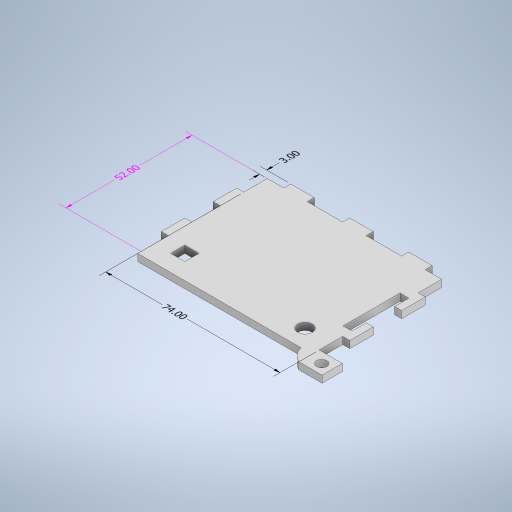
# Autodesk Inventor part: Parede_lateral_2
Saved by Autodesk Inventor 2024 (Build 280153000, 153)
## iProperties
Created: 2023-11-29
Part Number: Parede_lateral_2
Material: Genérico
Document SubType Name: Modeling
Designer: caiot
Density: 1 g/cm^3
Appearance: Padrão
Author: caiot
Autodesk Inventor part; units mm, degrees
ref_plane "YZ Plane" through (0, 0, 0) normal (1, 0, 0) x (0, 1, 0)
ref_plane "XZ Plane" through (0, 0, 0) normal (0, 1, 0) x (-1, 0, 0)
ref_plane "XY Plane" through (0, 0, 0) normal (0, 0, 1) x (1, 0, 0)
sketch "Esboço1" plane through (0, 0, 0) normal (0, 1, 0) x (-1, 0, 0)
  line L0 (0, 0) -> (-74, 0)
  line L1 (-74, 0) -> (-74, -52)
  line L2 (-74, -52) -> (0, -52)
  line L3 (0, -52) -> (0, 0)
  line L4 (-6.0465, -39.0348) -> (-22.7965, -39.0348)
  line L5 (-22.7965, -39.0348) -> (-22.7965, -36.6698)
  line L6 (-22.7965, -36.6698) -> (-6.0465, -36.6698)
  line L7 (-6.0465, -36.6698) -> (-6.0465, -39.0348)
  dimension "d0" = 74
  dimension "d1" = 52
  dimension "d22" = 16.75
  dimension "d23" = 2.365
  constraints: 16 end point, 4 parallel, 2 horizontal, 2 perpendicular
  measures "d0" distance of L2.end L1.end
  measures "d1" distance of L1.end L0.end
  measures "d22" distance of L5.end L6.end
  measures "d23" distance of L4.end L5.end
extrude "Extrusão1" add sketch "Esboço1" along normal blind 3 contours L3 L2 L1 L0 | L4 L5 L6 L7
sketch "Esboço2" plane through (0, 3, 0) normal (0, 1, 0) x (1, 0, 0)
  line L0 (0, 52) -> (0, 0) projected
  line L1 (74, 52) -> (0, 52) projected
  line L2 (7, 52) -> (17, 52)
  line L3 (17, 52) -> (17, 55)
  line L4 (17, 55) -> (7, 55)
  line L5 (7, 55) -> (7, 52)
  line L6 (32, 52) -> (42, 52)
  line L7 (42, 52) -> (42, 55)
  line L8 (42, 55) -> (32, 55)
  line L9 (32, 55) -> (32, 52)
  line L10 (57, 52) -> (67, 52)
  line L11 (67, 52) -> (67, 55)
  line L12 (67, 55) -> (57, 55)
  line L13 (57, 55) -> (57, 52)
  line L14 (74, 0) -> (74, 52) projected
  point P0 (17, 52)
  point P1 (67, 52)
  point P2 (42, 52)
  point P3 (7, 53.5)
  point P4 (67, 53.5)
  point P5 (57, 53.5)
  point P6 (42, 53.5)
  point P7 (17, 53.5)
  point P8 (32, 53.5)
  point P9 (0, 26)
  dimension "d13" = 3
  dimension "d38" = 7
  dimension "d39" = 7
  dimension "d40" = 15
  dimension "d42" = 10
  dimension "d44" = 10
  dimension "d45" = 10
  constraints: 24 end point, 7 midpoint, 6 parallel, 5 point on line, 3 horizontal, 3 perpendicular
  measures "d13" distance of L3.end L2.end
  measures "d38" distance from line of L0 point (7, 53.5)
  measures "d39" distance from line of L14 point (67, 53.5)
  measures "d40" distance of point (57, 53.5) point (42, 53.5)
  measures "d42" distance from line of point (17, 53.5) L5
  measures "d44" distance of point (67, 53.5) point (57, 53.5)
  measures "d45" distance of point (32, 53.5) point (42, 53.5)
extrude "Extrusão2" add sketch "Esboço2" against normal blind 3
sketch "Esboço5" plane through (0, 3, 0) normal (0, 1, 0) x (1, 0, 0)
  circle A0 centre (63, 5) radius 3.1
  line L0 (0, 52) -> (0, 0) projected
  line L1 (7, 52) -> (0, 52) projected
  line L2 (74, 0) -> (74, 52) projected
  line L3 (0, 0) -> (74, 0) projected
  point P0 (3.5, 52)
  dimension "d46" = 6.2
  dimension "d113" = 11
  dimension "d114" = 52
  dimension "d116" = 5
  constraints: 1 centre point, 1 midpoint
  measures "d46" diameter of A0
  measures "d113" distance from line of L2 A0.centre
  measures "d114" distance from line of L3 point (3.5, 52)
  measures "d116" distance from line of L3 A0.centre
extrude "Extrusão4" cut sketch "Esboço5" against normal blind 10
sketch "Esboço6" plane through (0, 3, 0) normal (0, 1, 0) x (1, 0, 0)
  line L0 (70.25, 13.9187) -> (74, 13.9188)
  line L1 (74, 13.9188) -> (74, 38.0813)
  line L2 (74, 38.0813) -> (70.25, 38.0813)
  line L3 (70.25, 38.0813) -> (70.25, 13.9187)
  line L4 (74, 0) -> (74, 52) projected
  line L5 (74, 52) -> (67, 52) projected
  line L6 (0, 0) -> (74, 0) projected
  point P0 (72.125, 38.0813)
  dimension "d49" = 3.75
  dimension "d50" = 24.1625
  dimension "d51" = 0
  dimension "d55" = 13.9187
  dimension "d100" = 13.9187
  constraints: 8 end point, 2 parallel, 1 horizontal, 1 midpoint, 1 perpendicular
  measures "d49" distance of L2.end L1.end
  measures "d50" distance of L1.end L0.end
  measures "d51" distance between parallel lines of L4 L1
  measures "d55" distance from line of L5 point (72.125, 38.081)
  measures "d100" distance between parallel lines of L6 L0
extrude "Extrusão5" cut sketch "Esboço6" against normal blind 10
sketch "Esboço7" plane through (0, 3, 0) normal (0, 1, 0) x (1, 0, 0)
  line L0 (0, 10) -> (-3, 10)
  line L1 (-3, 10) -> (-3, 20)
  line L2 (-3, 20) -> (0, 20)
  line L3 (0, 20) -> (0, 10)
  line L4 (0, 42) -> (-3, 42)
  line L5 (-3, 42) -> (-3, 32)
  line L6 (-3, 32) -> (0, 32)
  line L7 (0, 32) -> (0, 42)
  line L8 (7, 52) -> (0, 52) projected
  line L9 (0, 0) -> (74, 0) projected
  line L10 (74, 10) -> (77, 10)
  line L11 (77, 10) -> (77, 20)
  line L12 (77, 20) -> (74, 20)
  line L13 (74, 20) -> (74, 10)
  line L14 (74, 52) -> (67, 52) projected
  line L15 (74, 38.0813) -> (74, 52) projected
  line L16 (74, 42) -> (77, 42)
  line L17 (77, 42) -> (77, 32)
  line L18 (77, 32) -> (74, 32)
  line L19 (74, 32) -> (74, 42)
  line L20 (0, 0) -> (74, 0) projected
  point P0 (-1.5, 42)
  point P1 (7, 0)
  point P2 (-1.5, 10)
  point P3 (75.5, 42)
  point P4 (67, 0)
  point P5 (37, 0)
  point P6 (75.5, 10)
  dimension "d66" = 3
  dimension "d67" = 10
  dimension "d68" = 3
  dimension "d69" = 10
  dimension "d70" = 10
  dimension "d71" = 10
  dimension "d74" = 3
  dimension "d76" = 3
  dimension "d77" = 10
  dimension "d78" = 10
  dimension "d81" = 10
  constraints: 32 end point, 8 parallel, 5 midpoint, 4 horizontal, 4 perpendicular, 2 point on line
  measures "d66" distance of L1.end L2.end
  measures "d67" distance of L0.end L1.end
  measures "d68" distance of L6.end L5.end
  measures "d69" distance of L5.end L4.end
  measures "d70" distance from line of point (-1.5, 42) L8
  measures "d71" distance from line of L9 point (-1.5, 10)
  measures "d74" distance of L12.end L11.end
  measures "d76" distance of L17.end L18.end
  measures "d77" distance of L16.end L17.end
  measures "d78" distance from line of L14 point (75.5, 42)
  measures "d81" vertical distance of point (37, 0) point (75.5, 10)
extrude "Extrusão6" add sketch "Esboço7" against normal blind 3
sketch "Esboço8" plane through (0, 0, 0) normal (0, -1, 0) x (1, 0, 0)
  line L0 (0, 0) -> (74, 0) projected
  line L1 (69, 0) -> (83.8454, 0)
  line L2 (83.8454, 0) -> (83.8454, 8.6)
  line L3 (74, 0) -> (74, -10) projected
  circle A0 centre (79.548, 4.45) radius 2.2
  line L4 (74, 0) -> (74, 8.6)
  arc A1 (74, 8.6) -> (69, 0) centre (77.4588, 0.8356) ccw
  line L5 (74, 8.6) -> (83.8454, 8.6)
  point P0 (83.8454, 4.3)
  point P1 (74, 4.3)
  dimension "d84" = 8.6
  dimension "d86" = 4.4
  dimension "d94" = 8.5
  dimension "d99" = 5
  dimension "d101" = 4.15
  dimension "d104" = 5.55
  dimension "d106" = 4.3
  constraints: 8 end point, 2 centre point, 2 horizontal, 2 midpoint, 2 point on circle, 1 perpendicular, 1 point on line
  measures "d84" distance of L2.end L1.end
  measures "d86" diameter of A0
  measures "d94" radius of A1
  measures "d99" distance from line of L1.start L4
  measures "d101" distance from line of L5 A0.centre
  measures "d104" distance of point (74, 4.3) A0.centre
  measures "d106" distance of point (83.845, 4.3) A0.centre
extrude "Extrusão7" add sketch "Esboço8" against normal blind 3
sketch "Esboço10" plane through (0, 0, 0) normal (0, -1, 0) x (1, 0, 0)
  line L0 (83.8454, 0) -> (74, 0) projected
  line L1 (74, 0) -> (0, 0)
  line L2 (0, 0) -> (0, 3)
  line L3 (0, 3) -> (74, 3)
  line L4 (74, 3) -> (74, 0)
  dimension "d95" = 3
  constraints: 8 end point, 2 parallel, 1 horizontal, 1 perpendicular
  measures "d95" distance of L1.end L2.end
extrude "Extrusão9" add sketch "Esboço10" against normal blind 3
sketch "Esboço11" plane through (0, 3, 0) normal (0, 1, 0) x (1, 0, 0)
  line L0 (13, 4) -> (7, 4)
  line L1 (7, 4) -> (7, 10)
  line L2 (7, 10) -> (13, 10)
  line L3 (13, 10) -> (13, 4)
  line L4 (0, 10) -> (0, -3) projected
  line L5 (0, -3) -> (69.239, -3) projected
  line L6 (-3, 10) -> (0, 10) projected
  point P0 (0, 0)
  dimension "d107" = 6
  dimension "d108" = 6
  dimension "d109" = 7
  dimension "d115" = 0
  constraints: 8 end point, 2 parallel, 1 horizontal, 1 perpendicular
  measures "d107" distance of L1.end L2.end
  measures "d108" distance of L0.end L1.end
  measures "d109" distance between parallel lines of L4 L1
  measures "d115" distance between parallel lines of L6 L2
extrude "Extrusão10" cut sketch "Esboço11" against normal blind 10
equation "\"d40\" = d12"
equation "\"d12\" = 15"
